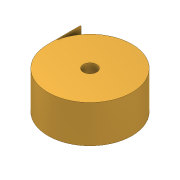
# Autodesk Inventor part: CF Spring with hole
Saved by Autodesk Inventor 2021.3 (Build 253353000, 353)
## iProperties
Created: 2022-06-28
Part Number: CF Spring with hole
Material: Generic
Document SubType Name: Modeling
Designer: david
Density: 1 g/cm^3
Appearance: Brass - Satin
Author: david
Autodesk Inventor part; units mm, degrees
ref_plane "YZ Plane" through (0, 0, 0) normal (1, 0, 0) x (0, 1, 0)
ref_plane "XZ Plane" through (0, 0, 0) normal (0, 1, 0) x (-1, 0, 0)
ref_plane "XY Plane" through (0, 0, 0) normal (0, 0, 1) x (1, 0, 0)
sketch "Sketch1" plane through (0, 0, 0) normal (0, 1, 0) x (-1, 0, 0)
  arc A0 (15.625, 0) -> (15.325, -3.0471) centre (0, 0) ccw
  circle A1 centre (0, 0) radius 2.5
  line L0 (15.625, 0) -> (15.625, -12)
  line L1 (15.625, -12) -> (15.325, -12)
  line L2 (15.325, -12) -> (15.325, -3.0471)
  dimension "d0" = 31.25
  dimension "d1" = 5
  dimension "d4" = 0.3
  dimension "d5" = 12
  constraints: 6 end point, 2 centre point, 2 coincident, 2 point on circle, 1 horizontal, 1 perpendicular, 1 tangent, 1 vertical
  measures "d0" diameter of A0
  measures "d1" diameter of A1
  measures "d4" distance of L0.end L1.end
  measures "d5" distance of L0.start L0.end
extrude "Extrusion1" add sketch "Sketch1" along normal blind 14
sketch "Sketch2" plane through (-15.625, 0, -12) normal (-1, 0, 0) x (0, 0, 1)
  point P0 (12, 0)
  point P1 (5.1198, 6.8941)
hole "Hole1" at (-15.625, 6.8941, -6.8802) direction (1, 0, 0) diameter 6.15 depth 0.3
body "Solid1"
